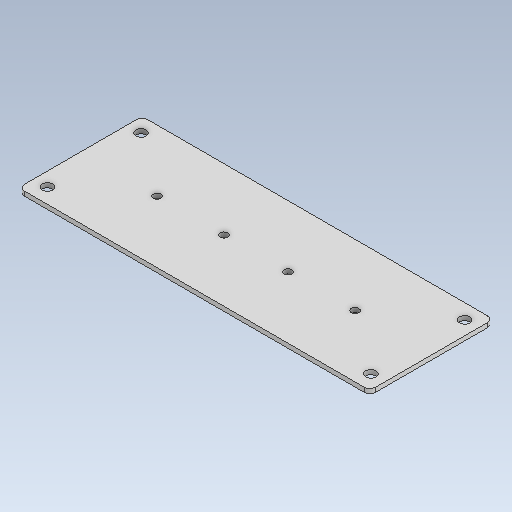
# Autodesk Inventor part: Interstage A
Saved by Autodesk Inventor 2020.3 (Build 243373000, 373)
## iProperties
Created: 2020-05-18
Part Number: Interstage A
Material: Genérico
Document SubType Name: Modeling
Designer: javic
Density: 1 g/cm^3
Appearance: Valor por defecto
Mass: 2.45575 g
Surface Area: 50.0845 cm^2
Volume: 2.45575 cm^3
Author: javic
Autodesk Inventor part; units mm, degrees
ref_plane "YZ Plane" through (0, 0, 0) normal (1, 0, 0) x (0, 1, 0)
ref_plane "XZ Plane" through (0, 0, 0) normal (0, 1, 0) x (-1, 0, 0)
ref_plane "XY Plane" through (0, 0, 0) normal (0, 0, 1) x (1, 0, 0)
sketch "Boceto1" plane through (0, 0, 0) normal (0, 1, 0) x (-1, 0, 0)
  arc A0 (-1.27, 1.27) -> (0, 0) centre (0, 1.27) ccw
  line L0 (0, 0) -> (79.96, 0)
  arc A1 (79.96, 0) -> (81.23, 1.27) centre (79.96, 1.27) ccw
  line L1 (81.23, 1.27) -> (81.23, 27.73)
  arc A2 (81.23, 27.73) -> (79.96, 29) centre (79.96, 27.73) ccw
  line L2 (79.96, 29) -> (0, 29)
  arc A3 (0, 29) -> (-1.27, 27.73) centre (0, 27.73) ccw
  line L3 (-1.27, 27.73) -> (-1.27, 1.27)
  circle A4 centre (77.98, 3.5) radius 1.25
  circle A5 centre (1.98, 25.5) radius 1.25
  circle A6 centre (1.98, 3.5) radius 1.25
  circle A7 centre (77.98, 25.5) radius 1.25
  circle A8 centre (47.48, 14.5) radius 0.9
  circle A9 centre (32.48, 14.5) radius 0.9
  point P0 (0, 0)
  constraints: 10 centre point, 8 end point, 8 point on circle, 8 tangent, 7 equal radius, 2 perpendicular, 1 parallel
extrude "Extrusión1" add sketch "Boceto1" along normal blind 1.04
sketch "Boceto3" plane through (0, 1.04, 0) normal (0, 1, 0) x (1, 0, 0)
  circle A0 centre (-63.23, -14.5) radius 0.9
  circle A1 centre (-16.73, -14.5) radius 0.9
  line L0 (-81.23, -1.27) -> (-81.23, -27.73) projected
  line L1 (0, 0) -> (-79.96, 0) projected
  line L2 (1.27, -27.73) -> (1.27, -1.27) projected
  line L3 (-79.96, -29) -> (0, -29) projected
  dimension "d15" = 1.8
  dimension "d16" = 1.8
  dimension "d17" = 18
  dimension "d18" = 14.5
  dimension "d19" = 18
  dimension "d20" = 14.5
  constraints: 2 centre point
  measures "d15" diameter of A0
  measures "d16" diameter of A1
  measures "d17" distance from line of L0 A0.centre
  measures "d18" distance from line of L1 A0.centre
  measures "d19" distance from line of L2 A1.centre
  measures "d20" distance from line of L3 A1.centre
hole "Agujero2" at (-63.23, 1.04, 14.5) at (-16.73, 1.04, 14.5) direction (0, -1, 0) diameter 1.8 end through all
